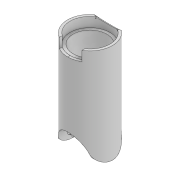
# Autodesk Inventor part: Socket_v2
Saved by Autodesk Inventor 2020 (Build 240168000, 168)
## iProperties
Created: 2021-03-25
Part Number: Socket_v2
Material: Generic
Document SubType Name: Modeling
Designer: deox
Density: 1 g/cm^3
Appearance: Default
Author: deox
Autodesk Inventor part; units mm, degrees
ref_plane "YZ Plane" through (0, 0, 0) normal (1, 0, 0) x (0, 1, 0)
ref_plane "XZ Plane" through (0, 0, 0) normal (0, 1, 0) x (-1, 0, 0)
ref_plane "XY Plane" through (0, 0, 0) normal (0, 0, 1) x (1, 0, 0)
sketch "Sketch1" plane through (0, 0, 0) normal (0, 0, 1) x (1, 0, 0)
  line L0 (0, 0) -> (10.33, 0)
  line L1 (8.133, 28.571) -> (8.133, 26.271)
  line L2 (8.133, 26.271) -> (6.933, 26.271)
  line L3 (10.33, 0) -> (9.2116, 0)
  line L4 (0, 0) -> (0, 4.8929)
  line L5 (8.133, 28.571) -> (6.633, 28.571)
  line L6 (6.633, 28.571) -> (6.633, 30.501)
  line L7 (6.633, 30.501) -> (9.133, 30.501)
  line L8 (9.133, 30.501) -> (10.333, 30.501) construction
  line L9 (10.333, 30.501) -> (10.33, 26.501) construction
  line L10 (10.33, 26.501) -> (9.133, 30.501)
  line L11 (10.33, 26.501) -> (10.33, 0)
  line L12 (9.2116, 0) -> (9.2116, 24.534) construction
  line L13 (9.2116, 24.534) -> (10.33, 24.534)
  line L14 (10.33, 24.534) -> (8.88, 24.534)
  line L15 (8.88, 24.534) -> (8.5253, 24.534)
  arc A0 (8.5253, 24.534) -> (6.933, 26.271) centre (4.9777, 22.8803) ccw
  line L16 (10.33, 0) -> (10.33, -10)
  line L17 (10.33, -10) -> (9.2116, -10)
  line L18 (9.2116, 0) -> (9.2116, -10)
  line L19 (10.33, 24.534) -> (8.133, 24.534)
  line L20 (8.133, 26.271) -> (8.133, 23.9355)
  arc A1 (8.133, 24.534) -> (6.933, 26.271) centre (2.7329, 22.0864) ccw
  line L21 (10.33, 0) -> (8.33, 0)
  line L22 (0, 0) -> (9, 0)
  line L23 (8.133, 28.571) -> (8.133, 32.1643)
  line L24 (9.133, 30.501) -> (9.133, 24.534)
  line L25 (9.133, 30.501) -> (15.1, 30.501) construction
  line L26 (8.133, 24.534) -> (8.133, 0)
  line L27 (6.933, 26.271) -> (6.933, 0)
  line L28 (6.933, 26.271) -> (33.204, 26.271) construction
  arc A2 (9.133, 24.534) -> (9.133, 30.501) centre (-13.3369, 27.5175) ccw
  line L29 (9.133, 24.534) -> (9.133, 0)
  line L30 (9.133, 24.534) -> (33.667, 24.534) construction
  line L31 (6.933, 0) -> (6.933, -10)
  line L32 (9.133, 0) -> (9.133, -10)
  line L33 (9.133, -10) -> (6.933, -10)
  dimension "d0" = 10.33
  dimension "d10" = 2.3
  dimension "d11" = 1.2
  dimension "d12" = 1.1184
  dimension "d20" = 1.5
  dimension "d21" = 1.93
  dimension "d22" = 2.5
  dimension "d23" = 1.2
  dimension "d24" = 4
  dimension "d25" = 24.534
  dimension "d27" = 0.3547
  dimension "d46" = 10
  dimension "d69" = 2
  dimension "d70" = 9
  dimension "d71" = 90
  dimension "d72" = 90
  dimension "d73" = 90
  dimension "d74" = 10
  dimension "d75" = 10
  constraints: 68 end point, 13 perpendicular, 12 point on line, 6 horizontal, 6 point on circle, 5 vertical, 3 centre point
  measures "d0" distance of L0.end L0.start
  measures "d10" distance of L1.start L1.end
  measures "d11" distance of L1.end L2.end
  measures "d12" distance of L0.end L3.end
  measures "d20" distance of L1.start L5.end
  measures "d21" distance of L5.end L6.end
  measures "d22" distance of L6.end L7.end
  measures "d23" distance of L7.end L8.end
  measures "d24" distance of L8.end L9.end
  measures "d25" distance of L3.end L12.end
  measures "d27" distance of L14.end L15.end
  measures "d46" distance of L0.end L16.end
  measures "d69" distance of L0.end L21.end
  measures "d70" distance of L0.start L22.end
  measures "d71" angle of L24 L25
  measures "d72" angle of L27 L28
  measures "d73" angle of L29 L30
  measures "d74" distance of L27.end L31.end
  measures "d75" distance of L29.end L32.end
revolve "Revolution1" add sketch "Sketch1" angle 360 about axis through (0, 0, 0) along (0, 1, 0) contours L27 A1 L20 L26 L0 | L0 L32 L33 L31 | L26 L20 L19 L15 L14 L29 L0 | L2 L20 A0 | A0 L20 A1 | L1 L23 L7 L24 L14 L15 A0 L20 | A0 L19 L20 | L5 L6 L7 L23
sketch "Sketch2" plane through (0, 0, 0) normal (0, 0, 1) x (1, 0, 0)
  line L0 (-6.633, 30.501) -> (6.633, 30.501) projected
  line L1 (-9.133, 30.501) -> (9.133, 30.501) projected
  line L2 (0, 30.501) -> (-4.6, 30.501)
  line L3 (-4.6, 30.501) -> (-4.6, 26.511)
  line L4 (-4.6, 26.511) -> (0, 26.501)
  line L5 (-10.33, 26.501) -> (10.33, 26.501) projected
  line L6 (0, 30.501) -> (0, 31.8797)
  line L7 (0, 30.501) -> (4.6, 30.501)
  line L8 (4.6, 30.501) -> (4.6, 26.511)
  line L9 (4.6, 26.511) -> (0, 26.501)
  point P0 (0, 0)
  point P1 (4.6, 29.647)
  dimension "d28" = 4.6
  dimension "d29" = 3.99
  constraints: 14 end point, 2 midpoint, 2 symmetric about line, 1 perpendicular, 1 point on line, 1 vertical
  measures "d28" distance of L2.start L2.end
  measures "d29" distance of L2.end L3.end
extrude "Extrusion1" cut sketch "Sketch2" along normal blind 12.5
sketch "Sketch4" plane through (0, 0, 0) normal (0, 0, 1) x (1, 0, 0)
  line L0 (-6.633, 30.501) -> (6.633, 30.501) projected
  line L1 (0, 30.501) -> (-4.6, 30.501)
  line L2 (-4.6, 30.501) -> (-4.6, 29.881)
  line L3 (-4.6, 30.501) -> (-4.6, 28.571) projected
  line L4 (-4.6, 29.881) -> (0, 29.881)
  line L5 (0, 30.501) -> (0, 31.4354)
  line L6 (0, 30.501) -> (4.6, 30.501)
  line L7 (4.6, 30.501) -> (4.6, 29.881)
  line L8 (4.6, 29.881) -> (0, 29.881)
  point P0 (0, 0)
  dimension "d32" = 4.6
  dimension "d33" = 0.62
  constraints: 14 end point, 1 collinear, 1 midpoint, 1 perpendicular, 1 point on line, 1 symmetric about line, 1 vertical
  measures "d32" distance of L1.start L1.end
  measures "d33" distance of L1.end L2.end
extrude "Extrusion3" cut sketch "Sketch4" against normal blind 12.5
sketch "Sketch5" plane through (0, 29.881, 0) normal (0, 1, 0) x (1, 0, 0)
  line L0 (0.256, 9.2303) -> (-0.256, 9.2303)
  line L1 (-0.256, 9.2303) -> (-0.256, 9.4068)
  line L2 (-0.256, 9.4068) -> (0.256, 9.4068)
  line L3 (0.256, 9.4068) -> (0.256, 9.2303)
  arc A0 (4.6, 8.104) -> (-4.6, 8.104) centre (0, 0) ccw projected
  line L4 (0.256, 9.2303) -> (-0.256, 9.4068) construction
  line L5 (-0.256, 9.2303) -> (0.256, 9.4068) construction
  point P0 (0, 9.3185)
  constraints: 12 end point, 2 midpoint, 2 parallel, 1 horizontal, 1 perpendicular, 1 point on circle
extrude "Extrusion4" cut sketch "Sketch5" against normal blind 0.01
sketch "Sketch7" plane through (0, 0, 0) normal (1, 0, 0) x (0, 1, 0)
  line L0 (28.571, -6.633) -> (29.881, -6.633) projected
  line L1 (29.8802, -4.7788) -> (29.4475, -8.2529) projected
  line L2 (29.881, -6.633) -> (29.5571, -7.3732)
  line L3 (29.2928, -9.4945) -> (26.501, -10.33) projected
  line L4 (26.501, -10.33) -> (27.868, -9.9209)
  arc A0 (29.5571, -7.3732) -> (27.868, -9.9209) centre (48.0947, -21.4969) ccw
  circle A1 centre (48.0947, -21.4969) radius 23.305
  line L5 (48.0947, 1.8081) -> (48.0947, -44.8018)
  point P0 (0, 0)
  point P1 (29.4475, -8.2529)
  dimension "d43" = 0.808
  dimension "d44" = 1.4269
  constraints: 6 end point, 5 point on circle, 2 centre point, 1 coincident, 1 point on line, 2 other
  measures "d43" distance of L0.end L2.end
  measures "d44" distance of L3.end L4.end
revolve "Revolution2" cut sketch "Sketch7" angle 360 about axis through (0, 48.0947, 1.8081) along (0, 0, -1) contours A1 L5 A0
sketch "Sketch8" plane through (0, 0, 0) normal (0, 0, 1) x (1, 0, 0)
  line L0 (-9.2116, -10) -> (9.2116, -10) projected
  ellipse E0 centre (0, -10) end of major axis (9.2116, -10) minor radius 10
  line L1 (6.933, -10) -> (6.933, 26.271) projected
  line L2 (-6.933, -10) -> (6.933, -10) projected
  ellipse E1 centre (0, -10) end of major axis (0, 0) minor radius 6.933
  point P0 (0, 0)
  constraints: 1 coincident, 1 horizontal, 1 midpoint, 8 other
extrude "Extrusion6" cut sketch "Sketch8" against normal mid plane 46.75 contours E1 L0 picked at (2.2728, -8.5153)
sketch "Sketch9" plane through (0, 0, 0) normal (1, 0, 0) x (0, 1, 0)
  line L0 (0, 6.933) -> (-10, 0) projected
  ellipse E0 centre (-4.8407, 0) end of major axis (-10, 0) minor radius 6.7445
  line L1 (-5.9852, 6.5764) -> (-11.2874, 6.5764)
  line L2 (-11.2874, 6.5764) -> (-11.2874, 0)
  line L3 (-11.2874, 0) -> (-10.5929, 0)
  line L4 (-5.9852, -6.5764) -> (-11.2874, -6.5764)
  line L5 (-11.2874, -6.5764) -> (-11.2874, 0)
  point P0 (0, 0)
  constraints: 10 end point, 2 perpendicular, 2 symmetric about line, 1 horizontal, 4 other
extrude "Extrusion7" cut sketch "Sketch9" against normal mid plane 46.75 contours E0 L4 L5 L2 L1
sketch "Sketch10" plane through (0, 0, 0) normal (1, 0, 0) x (0, 1, 0)
  circle A0 centre (-5.5646, 0) radius 1.2
  point P0 (0, 0)
  dimension "d51" = 2.4
  constraints: 1 centre point
  measures "d51" diameter of A0
extrude "Extrusion8" add sketch "Sketch10" along normal blind 8.75 and the other way blind 8.875
sketch "Sketch11" plane through (0, 0, 0) normal (1, 0, 0) x (0, 1, 0)
  spline S0 degree 2 poles (-4.3646, 0) (-4.3646, -2.0785) (-6.1646, -1.0392) (-7.9646, 0) (-6.1646, 1.0392) (-4.3646, 2.0785) (-4.3646, 0) knots 0 0 0 0.333333 0.333333 0.666667 0.666667 1 1 1 weights 1 0.5 1 0.5 1 0.5 1 projected
  point P0 (0, 0)
  constraints: 1 other
extrude "Extrusion9" cut sketch "Sketch11" against normal mid plane 11.75
ref_plane "Work Plane2" through (0, -5.5646, 0) normal (1, 0, 0) x (0, 0, -1)
sketch "Sketch13" plane through (0, -5.5646, 0) normal (1, 0, 0) x (0, 0, -1)
  circle A0 centre (0, 0) radius 3
  circle A1 centre (0, 0) radius 1.2 projected
  point P0 (0, 5.5646)
  dimension "d61" = 6
  constraints: 1 centre point
  measures "d61" diameter of A0
extrude "Extrusion11" cut sketch "Sketch13" against normal mid plane 14
sketch "Sketch14" plane through (0, 26.271, 0) normal (0, 1, 0) x (1, 0, 0)
  circle A0 centre (0, 0) radius 6.933 projected
  circle A1 centre (0, 0) radius 8.133 projected
extrude "Extrusion12" cut sketch "Sketch14" along normal blind 10 contours A0 | A1
sketch "Sketch16" plane through (0, 26.271, 0) normal (0, 1, 0) x (1, 0, 0)
  circle A0 centre (0, 0) radius 6.933 projected
  circle A1 centre (0, 0) radius 8.133 projected
extrude "Extrusion14" add sketch "Sketch16" along normal blind 0.25
body "Solid1"
